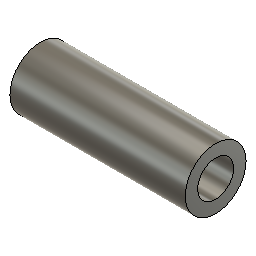
pipe v1 (Autodesk Fusion 360 design; units mm, degrees)
Autodesk Fusion 360 part; units mm, degrees
sketch "Sketch1" plane through (0, 0, 0) normal (0, 0, 1) x (1, 0, 0)
  line L0 (-10.8538, 4.3293) -> (31.4462, 4.3293)
  line L1 (31.4462, 4.3293) -> (31.4462, 7.3293)
  line L2 (31.4462, 7.3293) -> (-10.8538, 7.3293)
  line L3 (-10.8538, 7.3293) -> (-10.8538, 4.3293)
  line L4 (10.2962, 7.3293) -> (10.2962, 4.3293) construction
  line L5 (31.4462, 5.8293) -> (-10.8538, 5.8293) construction
  line L6 (9.2962, 4.3293) -> (11.2962, 4.3293)
  line L7 (11.2962, 4.3293) -> (11.2962, 4.0293)
  line L8 (11.2962, 4.0293) -> (9.2962, 4.0293)
  line L9 (9.2962, 4.0293) -> (9.2962, 4.3293)
  line L10 (10.2962, 4.3293) -> (10.2962, 4.0293) construction
  dimension "d1" = 3
  dimension "d2" = 42.3
  dimension "d3" = 0.3
  dimension "d4" = 2
  measures "d2" distance of L1 L3
revolve "Revolve2" add sketch "Sketch1" angle 360 about axis through (1.75, 0, 0) along (1, 0, 0) contours L0 L1 L2 L3 L6 makes body 1
revolve "Revolve1" add sketch "Sketch1" angle 360 about axis through (1.75, 0, 0) along (1, 0, 0) separate body contours L0 L6 L7 L8 L9 makes body 2
sketch "Sketch2" plane through (31.4462, 0, 0) normal (1, 0, 0) x (0, 0, -1)
  circle A0 centre (0, 0) radius 7.3293
  circle A1 centre (0, 0) radius 4.3293
